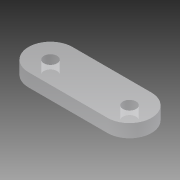
# Autodesk Inventor part: plastic_part_5
Saved by Autodesk Inventor 2013 (Build 170138000, 138)
## iProperties
Shininess: 20.0
Created: 2011-05-15
Part Number: plastic_part_5
Document SubType Name: Modeling
Designer: Noa Izumi
Material: Default
Density: 1 g/cm^3
Density: 0.0
Volumn: 0.0
Area: 0.0
PropertySet Name: Model Information
Control State: 0
Master: False
Checked Out: False
Author: Noa Izumi
Autodesk Inventor part; units mm, degrees
ref_plane "YZ Plane" through (0, 0, 0) normal (1, 0, 0) x (0, 1, 0)
ref_plane "XZ Plane" through (0, 0, 0) normal (0, 1, 0) x (-1, 0, 0)
ref_plane "XY Plane" through (0, 0, 0) normal (0, 0, 1) x (1, 0, 0)
sketch "Sketch1" plane through (0, 0, 0) normal (0, 0, 1) x (1, 0, 0)
  line L0 (5, -3) -> (23, -3)
  line L1 (28, 2) -> (28, 2)
  line L2 (23, 7) -> (5, 7)
  line L3 (0, 2) -> (0, 2)
  arc A0 (5, 7) -> (0, 2) centre (5, 2) ccw
  arc A1 (0, 2) -> (5, -3) centre (5, 2) ccw
  arc A2 (28, 2) -> (23, 7) centre (23, 2) ccw
  arc A3 (23, -3) -> (28, 2) centre (23, 2) ccw
  circle A4 centre (5, 2) radius 1.5
  circle A5 centre (23, 2) radius 1.5
  point P0 (0, -3)
  point P1 (28, -3)
  point P2 (0, 7)
  dimension "d0" = 28
  dimension "d1" = 10
  dimension "d2" = 5
  dimension "d4" = 3
  dimension "d5" = 3
  constraints: 8 end point, 8 point on circle, 8 tangent, 6 centre point, 6 point on line, 3 equal radius, 2 coincident, 2 parallel, 1 horizontal, 1 perpendicular
  measures "d0" distance of point (0, -3) point (28, -3)
  measures "d1" distance of point (0, 7) point (0, -3)
  measures "d2" radius of A0
  measures "d4" diameter of A5
  measures "d5" diameter of A4
extrude "Extrusion1" add sketch "Sketch1" along normal blind 3
